cable_clip (Autodesk Fusion 360 design; units mm, degrees)
Autodesk Fusion 360 part; units mm, degrees
note: some values were not read from the file. Set by a fixed rule: which sketch regions a step uses.
sketch "Sketch1" plane through (0, 0, 0) normal (0, 0, 1) x (1, 0, 0)
  line L0 (10, -2.5) -> (10, -4)
  line L1 (10, -4) -> (4, -4)
  line L2 (4, -4) -> (4, -6.6)
  line L3 (4, -6.6) -> (6, -6.6)
  line L4 (6, -6.6) -> (6, -9.1)
  line L5 (6, -9.1) -> (2.5, -9.1)
  line L6 (2.5, -9.1) -> (2.5, -4.0389)
  line L7 (-2.5, -4.0389) -> (-2.5, -9.1)
  line L8 (-2.5, -9.1) -> (-6, -9.1)
  line L9 (-6, -9.1) -> (-6, -6.6)
  line L10 (-6, -6.6) -> (-4, -6.6)
  line L11 (-4, -6.6) -> (-4, -4)
  line L12 (-4, -4) -> (-10, -4)
  line L13 (-10, -4) -> (-10, -2.5)
  line L14 (-10, -2.5) -> (-5.75, -2.5)
  line L15 (5.75, -2.5) -> (10, -2.5)
  arc A0 (2.5, -4.0389) -> (-2.5, -4.0389) centre (0, 0) ccw
  arc A1 (5.75, 0) -> (-5.75, 0) centre (0, 0) ccw
  line L16 (-5.75, 0) -> (-5.75, -2.5)
  line L17 (5.75, 0) -> (5.75, -2.5)
  dimension "d3" = 8
  dimension "d4" = 4
  dimension "d5" = 5
  dimension "d6" = 2.5
  dimension "d7" = 2.5
  dimension "d8" = 2.6
  dimension "d9" = 12
  dimension "d10" = 20
  dimension "d11" = 6
  dimension "d12" = 10
  dimension "d14" = 2.5
  dimension "d19" = 9.5
  dimension "d24" = 1.5
  dimension "d25" = 11.5
  constraint horizontal L14
  constraint perpendicular L0 L14
  constraint perpendicular L0 L1
  constraint perpendicular L1 L2
  constraint perpendicular L2 L3
  constraint perpendicular L3 L4
  constraint perpendicular L4 L5
  constraint perpendicular L5 L6
  constraint parallel L6 L7
  constraint perpendicular L7 L8
  constraint perpendicular L8 L9
  constraint perpendicular L7 L10
  constraint perpendicular L8 L11
  constraint perpendicular L11 L12
  constraint vertical L13
  constraint horizontal L1.end L11.end
  constraint horizontal L2.end L10.end
  constraint horizontal L5.end L7.end
  constraint collinear L14 L15
  constraint coincident A0.centre A1.centre
  constraint tangent A1 L16
  constraint tangent A1 L17
  constraint vertical L17
  constraint vertical L16
  measures "d3" distance of L2 L11
  measures "d4" distance of A0.centre L11
  measures "d5" distance of L6 L7
  measures "d6" distance of A0.centre L7
  measures "d7" distance of L8.end L9.end
  measures "d8" distance of L10.end L11.end
  measures "d9" distance of L4 L9
  measures "d10" distance of L0 L13
  measures "d11" distance of A0.centre L9
  measures "d12" distance of A0.centre L13
  measures "d14" vertical distance of A0.centre L0.start
  measures "d19" diameter of A0
  measures "d24" distance of L12.end L13.end
  measures "d25" diameter of A1
extrude "Extrude1" add sketch "Sketch1" along normal blind 10
chamfer "Chamfer1" distance 0.75 angle 45 4 edges at (-6, -6.6, 5) (-6, -9.1, 5) (6, -6.6, 5) (6, -9.1, 5)
fillet "Fillet3" radius 2 2 edges at (-5.75, -2.5, 5) (5.75, -2.5, 5)
equation "d4 = d3 / 2"
equation "d6 = d5 / 2"
equation "d11 = d9 / 2"
equation "d12 = d10 / 2"
